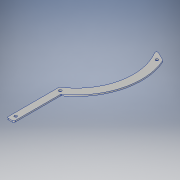
# Autodesk Inventor part: 2AM-17-P-5201 - claw arm
Saved by Autodesk Inventor 2017 (Build 210142000, 142)
## iProperties
Created: 2017-12-28
Part Number: 2AM-17-P-5201 - claw arm
Material: Aluminum 6061
Document SubType Name: Modeling
Designer: Micah
Density: 2.7 g/cm^3
Appearance: Aluminum - Flat
Author: Micah
Autodesk Inventor part; units mm, degrees
ref_plane "YZ Plane" through (0, 0, 0) normal (1, 0, 0) x (0, 1, 0)
ref_plane "XZ Plane" through (0, 0, 0) normal (0, 1, 0) x (-1, 0, 0)
ref_plane "XY Plane" through (0, 0, 0) normal (0, 0, 1) x (1, 0, 0)
sketch "Sketch1" plane through (0, 0, 0) normal (0, 1, 0) x (-1, 0, 0)
  line L0 (0, 0) -> (72.0519, -110.6962) construction
  line L1 (0, 0) -> (0, -132.08) construction
  arc A0 (-1.4091, -0.9301) -> (-42.2635, -176.856) centre (72.0519, -110.6962) ccw
  line L2 (72.0519, -110.6962) -> (-42.2635, -176.856) construction
  arc A1 (0, 22.1526) -> (-15.8725, 12.2248) centre (72.0519, -110.6962) ccw construction
  line L3 (0, 0) -> (-15.9623, 24.5235) construction
  line L4 (0, 1.7085) -> (0, 117.475)
  line L5 (-15.8725, 13.8467) -> (-15.8725, 117.475)
  line L6 (-3.175, 120.65) -> (-12.6975, 120.65)
  line L7 (-49.4275, -181.0021) -> (-64.4319, -173.8454)
  arc A2 (-17.173, 11.2841) -> (-65.9645, -172.2733) centre (72.0519, -110.6962) ccw
  line L8 (-42.2635, -176.856) -> (-41.282, -178.374)
  line L9 (-45.3151, -182.9636) -> (-49.4275, -181.0021)
  arc A3 (-45.3151, -182.9636) -> (-41.282, -178.374) centre (-43.9482, -180.0979) ccw
  arc A4 (-65.9645, -172.2733) -> (-64.4319, -173.8454) centre (-63.065, -170.9797) ccw
  arc A5 (-1.4091, -0.9301) -> (0, 1.7085) centre (-3.175, 1.7085) ccw
  arc A6 (-17.173, 11.2841) -> (-15.8725, 13.8467) centre (-19.0475, 13.8467) ccw
  arc A7 (0, 117.475) -> (-3.175, 120.65) centre (-3.175, 117.475) ccw
  arc A8 (-12.6975, 120.65) -> (-15.8725, 117.475) centre (-12.6975, 117.475) ccw
  point P0 (-65.4815, -173.3448)
  point P1 (0, 120.65)
  point P2 (-35.1928, -187.7917)
  dimension "d1" = 132.08
  dimension "d2" = 33.06
  dimension "d3" = 87
  dimension "d4" = 302.26
  dimension "d5" = 29.2608
  dimension "d6" = 120.65
  dimension "d8" = 3.175
  dimension "d9" = 3.175
  dimension "d10" = 3.175
  constraints: 22 point on circle, 20 end point, 12 tangent, 9 centre point, 8 point on line, 3 equal radius, 2 coincident, 1 collinear, 1 equal length
  measures "d1" distance of point (0, 0) L0.end
  measures "d2" angle of L1 L0
  measures "d3" angle of L0 L2
  measures "d4" diameter of A1
  measures "d5" distance of point (0, 0) L3.end
  measures "d6" distance of point (0, 0) point (0, 120.65)
  measures "d8" radius of A3
  measures "d9" radius of A4
  measures "d10" radius of A5
extrude "Extrusion1" add sketch "Sketch1" along normal blind 3.175
sketch "Sketch2" plane through (0, 3.175, 0) normal (0, 1, 0) x (1, 0, 0)
  arc A0 (17.173, -11.2841) -> (65.9645, 172.2733) centre (-72.0519, 110.6962) ccw projected
  line L0 (45.6255, 15.8684) -> (-72.0519, 110.6962)
  circle A1 centre (-72.0519, 110.6962) radius 151.13
  circle A2 centre (-72.0519, 110.6962) radius 132.0211
  circle A3 centre (-72.0519, 110.6962) radius 141.605
  circle A4 centre (57.9094, 166.9283) radius 3.175
  arc A5 (17.173, -11.2841) -> (15.8725, -13.8467) centre (19.0475, -13.8467) ccw projected
  line L1 (0, 0) -> (19.0475, -13.8467)
  circle A6 centre (8.2082, -5.967) radius 3.175
  line L2 (3.175, -120.65) -> (12.6975, -120.65) projected
  line L3 (7.9363, -120.65) -> (7.9363, 5.6655)
  circle A7 centre (7.9363, -107.95) radius 3.175
  dimension "d13" = 283.21
  dimension "d14" = 6.35
  dimension "d15" = 6.35
  dimension "d16" = 6.35
  dimension "d17" = 12.7
  constraints: 6 end point, 5 centre point, 3 point on circle, 2 coincident, 2 point on line, 1 concentric, 1 midpoint, 1 perpendicular, 3 other
  measures "d13" diameter of A3
  measures "d14" diameter of A4
  measures "d15" diameter of A6
  measures "d16" diameter of A7
  measures "d17" distance from line of L2 A7.centre
hole "Hole1" at (7.9363, 3.175, 107.95) at (8.2082, 3.175, 5.967) at (57.9094, 3.175, -166.9283) direction (0, -1, 0) diameter 6.35 depth 25.4 tip angle 118
body "Solid1"
